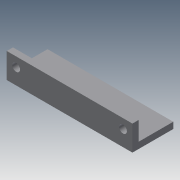
# Autodesk Inventor part: ruka_L
Saved by Autodesk Inventor 2013 (Build 170138000, 138)
## iProperties
Created: 2013-02-08
Part Number: ruka_L
Material: Generic
Document SubType Name: Modeling
Designer: idle-rug
Density: 1 g/cm^3
Author: idle-rug
Autodesk Inventor part; units mm, degrees
ref_plane "YZ Plane" through (0, 0, 0) normal (1, 0, 0) x (0, 1, 0)
ref_plane "XZ Plane" through (0, 0, 0) normal (0, 1, 0) x (-1, 0, 0)
ref_plane "XY Plane" through (0, 0, 0) normal (0, 0, 1) x (1, 0, 0)
sketch "Sketch1" plane through (0, 0, 0) normal (0, 1, 0) x (-1, 0, 0)
  line L0 (20, 3) -> (-20, 3)
  line L1 (-20, 3) -> (-20, -3)
  line L2 (-20, -3) -> (20, -3)
  line L3 (20, -3) -> (20, 3)
  line L4 (20, 3) -> (-20, -3) construction
  line L5 (-20, 3) -> (20, -3) construction
  point P0 (0, 0)
  dimension "d0" = 40
  dimension "d1" = 6
  constraints: 12 end point, 2 midpoint, 2 parallel, 1 horizontal, 1 perpendicular
  measures "d0" distance of L2.end L1.end
  measures "d1" distance of L1.end L0.end
extrude "Extrusion1" add sketch "Sketch1" along normal blind 2
sketch "Sketch3" plane through (0, 2, 0) normal (0, 1, 0) x (1, 0, 0)
  line L0 (20, -3) -> (20, 3) projected
  line L1 (20, 3) -> (-20, 3) projected
  line L2 (-20, 3) -> (-20, -3) projected
  line L3 (-20, 3) -> (-20, 1)
  line L4 (-20, 1) -> (20, 1)
  line L5 (20, 3) -> (20, 1)
  line L6 (-20, 3) -> (20, 3)
  point P0 (0, 0)
  dimension "d4" = 2
  constraints: 8 end point, 2 collinear, 2 point on line, 1 perpendicular
  measures "d4" distance of L1.end L3.end
extrude "Extrusion2" add sketch "Sketch3" along normal blind 11
sketch "Sketch4" plane through (-20, 0, 3) normal (0, 0, 1) x (1, 0, 0)
  line L0 (0, 0) -> (40, 0) projected
  line L1 (40, 0) -> (40, 2) projected
  line L2 (0, 2) -> (40, 2) projected
  line L3 (0, 0) -> (0, 2) projected
  point P0 (20, 0)
extrude "Extrusion3" add sketch "Sketch4" along normal blind 2
sketch "Sketch5" plane through (0, 2, 0) normal (0, 1, 0) x (1, 0, 0)
  line L0 (-20, -5) -> (-17, -5)
  line L1 (-17, -5) -> (-17, -2)
  line L2 (-17, -2) -> (-20, -2)
  line L3 (-20, -2) -> (-20, -5)
  circle A0 centre (-17, -2) radius 1.25
  line L4 (20, -5) -> (17, -5)
  line L5 (17, -5) -> (17, -2)
  line L6 (17, -2) -> (20, -2)
  line L7 (20, -2) -> (20, -5)
  circle A1 centre (17, -2) radius 1.25
  point P0 (0, 0)
  dimension "d9" = 3
  dimension "d10" = 2.5
  dimension "d11" = 3
  dimension "d12" = 3
  dimension "d13" = 2.5
  constraints: 16 end point, 4 parallel, 2 centre point, 2 coincident, 2 horizontal, 2 perpendicular
  measures "d9" distance of L2.end L1.end
  measures "d10" diameter of A0
  measures "d11" distance of L5.end L6.end
  measures "d12" distance of L4.end L5.end
  measures "d13" diameter of A1
extrude "Extrusion4" cut sketch "Sketch5" against normal blind 2 contours A0 L2 L1 | L1 L2 A0 | A1 L6 L5 | L5 L6 A1
body "Solid1"
